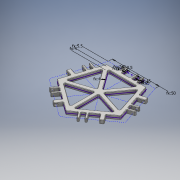
# Autodesk Inventor part: pentagon
Saved by Autodesk Inventor 2016 (Build 200138000, 138)
## iProperties
Created: 2016-11-12
Part Number: pentagon
Material: Generic
Document SubType Name: Modeling
Designer: Chris
Density: 1 g/cm^3
Appearance: Default
Author: Chris
Autodesk Inventor part; units mm, degrees
ref_plane "YZ Plane" through (0, 0, 0) normal (1, 0, 0) x (0, 1, 0)
ref_plane "XZ Plane" through (0, 0, 0) normal (0, 1, 0) x (-1, 0, 0)
ref_plane "XY Plane" through (0, 0, 0) normal (0, 0, 1) x (1, 0, 0)
sketch "Sketch1" plane through (0, 0, 0) normal (0, 0, 1) x (1, 0, 0)
  line L0 (25, 34.409548) -> (40.45085, -13.143278) construction
  line L1 (40.45085, -13.143278) -> (0, -42.53254) construction
  line L2 (0, -42.53254) -> (-40.45085, -13.143278) construction
  line L3 (-40.45085, -13.143278) -> (-25, 34.409548) construction
  line L4 (-25, 34.409548) -> (25, 34.409548) construction
  line L5 (21.004016, 28.909548) -> (33.985212, -11.042465)
  line L6 (33.985212, -11.042465) -> (0, -35.734167)
  line L7 (0, -35.734167) -> (-33.985212, -11.042465)
  line L8 (-33.985212, -11.042465) -> (-21.004016, 28.909548)
  line L9 (-21.004016, 28.909548) -> (21.004016, 28.909548)
  line L10 (0, -35.734167) -> (0, 0) construction
  line L11 (-18.097846, 24.909548) -> (-29.28293, -9.514601)
  line L12 (-29.28293, -9.514601) -> (0, -30.789895)
  line L13 (0, -30.789895) -> (29.28293, -9.514601)
  line L14 (29.28293, -9.514601) -> (18.097846, 24.909548)
  line L15 (18.097846, 24.909548) -> (-18.097846, 24.909548)
  line L16 (-7.5, 34.409548) -> (7.5, 34.409548) construction
  line L17 (3.475, 34.409548) -> (5.475, 34.409548) construction
  line L18 (5.475, 34.409548) -> (9.525, 34.409548) construction
  line L19 (11.525, 34.409548) -> (9.525, 34.409548) construction
  line L20 (-9.475, 34.409548) -> (-5.525, 34.409548) construction
  line L21 (-9.475, 28.909548) -> (-5.525, 28.909548)
  line L22 (-5.525, 28.909548) -> (-5.525, 36.409548)
  line L23 (-5.525, 36.409548) -> (-9.475, 36.409548)
  line L24 (-9.475, 36.409548) -> (-9.475, 28.909548)
  line L25 (3.475, 36.409548) -> (5.475, 36.409548)
  line L26 (5.475, 36.409548) -> (5.475, 28.909548)
  line L27 (5.475, 28.909548) -> (3.475, 28.909548)
  line L28 (3.475, 28.909548) -> (3.475, 36.409548)
  line L29 (9.525, 36.409548) -> (11.525, 36.409548)
  line L30 (11.525, 36.409548) -> (11.525, 28.909548)
  line L31 (11.525, 28.909548) -> (9.525, 28.909548)
  line L32 (9.525, 28.909548) -> (9.525, 36.409548)
  line L33 (-9.475, 34.409548) -> (-8.975, 34.409548)
  line L34 (-9.475, 34.409548) -> (-9.475, 35.909548)
  line L35 (-6.025, 34.409548) -> (-5.525, 34.409548)
  line L36 (-5.525, 34.409548) -> (-5.525, 35.909548)
  arc A0 (-8.975, 34.409548) -> (-9.475, 35.909548) centre (-11.475, 34.409548) ccw
  arc A1 (-5.525, 35.909548) -> (-6.025, 34.409548) centre (-3.525, 34.409548) ccw
  line L37 (5.475, 35.909548) -> (5.475, 34.409548)
  line L38 (5.475, 34.409548) -> (5.975, 34.409548)
  line L39 (9.525, 35.909548) -> (9.525, 34.409548)
  line L40 (9.525, 34.409548) -> (9.025, 34.409548)
  arc A2 (5.975, 34.409548) -> (5.475, 35.909548) centre (3.475, 34.409548) ccw
  arc A3 (9.525, 35.909548) -> (9.025, 34.409548) centre (11.525, 34.409548) ccw
  line L41 (-18.097846, 24.909548) -> (0, 0) construction
  line L42 (-29.28293, -9.514601) -> (0, 0) construction
  line L43 (18.097846, 24.909548) -> (0, 0) construction
  line L44 (29.28293, -9.514601) -> (0, 0) construction
  line L45 (0, 0) -> (-23.690388, 7.697474) construction
  line L46 (0, 24.909548) -> (0, 0) construction
  line L47 (0, 0) -> (23.690388, 7.697474) construction
  line L48 (0, 0) -> (14.641465, -20.152248) construction
  line L49 (-14.641465, -20.152248) -> (0, 0) construction
  line L50 (-18.861778, 22.558407) -> (-3.236068, 1.051462)
  line L51 (-3.236068, 1.051462) -> (-28.518998, -7.16346)
  line L52 (-15.62571, 24.909548) -> (0, 3.402603)
  line L53 (15.62571, 24.909548) -> (0, 3.402603)
  line L54 (18.861778, 22.558407) -> (3.236068, 1.051462)
  line L55 (28.518998, -7.16346) -> (3.236068, 1.051462)
  line L56 (27.28293, -10.967686) -> (2, -2.752764)
  line L57 (2, -2.752764) -> (2, -29.33681)
  line L58 (-2, -29.33681) -> (-2, -2.752764)
  line L59 (-2, -2.752764) -> (-27.28293, -10.967686)
  point P0 (0, 34.409548)
  dimension "d0" = 50
  dimension "d1" = 5.5
  dimension "d2" = 4
  dimension "d3" = 15
  dimension "d4" = 2
  dimension "d5" = 4.05
  dimension "d6" = 3.95
  dimension "d9" = 4
  dimension "d12" = 3
  dimension "d13" = 0.5
  dimension "d26" = 4
  constraints: 120 end point, 33 point on line, 16 parallel, 10 equal length, 9 midpoint, 8 horizontal, 8 point on circle, 7 coincident, 6 perpendicular, 5 vertical, 4 centre point, 2 collinear, 2 equal radius, 19 other
  measures "d0" distance of L3.end L0.start
  measures "d1" distance between parallel lines of L9 L4
  measures "d2" distance between parallel lines of L9 L15
  measures "d3" distance of L16.start L16.end
  measures "d4" distance of L19.start L18.end
  measures "d5" distance of L17.end L18.end
  measures "d6" distance of L20.start L20.end
  measures "d9" diameter of L23 L4
  measures "d12" diameter of L34.end L33
  measures "d13" distance of L20.start L33.end
  measures "d26" distance between parallel lines of L52 L50
extrude "Extrusion3" add sketch "Sketch1" along normal mid plane 4 contours L5 L6 L7 L8 L9 | L15 L52 L53 L14 L54 L55 L13 L56 L57 L12 L58 L59 L11 L51 L50
extrude "Extrusion2" add sketch "Sketch1" along normal mid plane 4 contours L9 L32 L29 L30 | L9 L28 L25 L26 | L24 L33 A0 L23 L22 A1 L35 L9 | L24 A0 L33 | L35 A1 L22
revolve "Revolution1" add sketch "Sketch1" angle 360 about axis through (-25, 34.409548, 0) along (1, 0, 0) contours L40 A3 L32 | L26 A2 L38
revolve "Revolution3" cut sketch "Sketch1" angle 360 about axis through (-9.475, 34.409548, 0) along (1, 0, 0) contours L24 A0 L33 | L35 A1 L22
fillet "Fillet5" radius 1 20 edges at (-21.004, 28.9095, 0) (21.004, 28.9095, 0) (33.9852, -11.0425, 0) (0, -35.7342, 0) (-33.9852, -11.0425, 0) (-18.8618, 22.5584, 0) (-15.6257, 24.9095, 0) (15.6257, 24.9095, 0) (0, 3.4026, 0) (-3.2361, 1.0515, 0) (-2, -2.7528, 0) (2, -2.7528, 0) (3.2361, 1.0515, 0) (-28.519, -7.1635, 0) (-27.2829, -10.9677, 0) (-2, -29.3368, 0) (2, -29.3368, 0) (27.2829, -10.9677, 0) (28.519, -7.1635, 0) (18.8618, 22.5584, 0)
pattern_circular "Circular Pattern1" count 5 over 360 about axis through (0, 0, -10) along (0, 0, 1) of "Extrusion2", "Revolution1", "Revolution3"
fillet "Fillet4" radius 0.75 60 edges at (-30.7249, -22.6817, 0) (-29.1069, -23.8573, 0) (-25.8304, -26.2378, 0) (-24.2123, -27.4134, 0) (-16.9312, -32.7035, 0) (-13.7356, -35.0252, 0) (29.0664, -23.8867, 0) (25.8708, -26.2084, 0) (18.5897, -31.4985, 0) (16.9716, -32.6741, 0) (13.6951, -35.0546, 0) (12.0771, -36.2302, 0) (38.189, 0.2902, 0) (37.5709, 2.1924, 0) (36.3194, 6.0441, 0) (35.7014, 7.9462, 0) (32.9202, 16.5058, 0) (31.6996, 20.2624, 0) (-9.475, 36.4095, 0) (-5.525, 36.4095, 0) (3.475, 36.4095, 0) (5.475, 36.4095, 0) (9.525, 36.4095, 0) (11.525, 36.4095, 0) (-31.6842, 20.31, 0) (-31.0661, 22.2121, 0) (-32.9357, 16.4582, 0) (-33.5537, 14.5561, 0) (-36.3349, 5.9966, 0) (-37.5555, 2.2399, 0) (-9.475, 28.9095, 0) (-5.525, 28.9095, 0) (3.475, 28.9095, 0) (5.475, 28.9095, 0) (9.525, 28.9095, 0) (11.525, 28.9095, 0) (24.5667, 17.9448, 0) (25.7873, 14.1881, 0) (28.5684, 5.6286, 0) (29.1865, 3.7265, 0) (30.438, -0.1253, 0) (31.056, -2.0274, 0) (24.658, -17.8191, 0) (21.4624, -20.1408, 0) (14.1813, -25.4309, 0) (12.5632, -26.6064, 0) (9.2867, -28.987, 0) (7.6687, -30.1625, 0) (-9.3272, -28.9576, 0) (-12.5228, -26.6358, 0) (-21.422, -20.1702, 0) (-19.8039, -21.3458, 0) (-26.3165, -16.6141, 0) (-24.6985, -17.7897, 0) (-30.4226, -0.0777, 0) (-29.2019, 3.679, 0) (-26.4208, 12.2385, 0) (-25.8027, 14.1406, 0) (-24.5512, 17.9924, 0) (-23.9332, 19.8945, 0)
chamfer "Chamfer2" distance 0.4 angle 45 260 edges at (-15.2512, 28.9095, 2) (-20.8653, 28.7186, 2) (-22.465, 24.4132, 2) (-24.0742, 20.1713, 2) (-27.4997, 21.0533, 2) (-30.9251, 21.9353, 2) (-31.3751, 21.261, 2) (-31.4074, 20.451, 2) (-28.1177, 19.1512, 2) (-24.828, 17.8513, 2) (-25.177, 16.0665, 2) (-25.9438, 14.4174, 2) (-29.3692, 15.2994, 2) (-32.7946, 16.1814, 2) (-33.2447, 15.5071, 2) (-33.2769, 14.6971, 2) (-29.9872, 13.3973, 2) (-26.6976, 12.0974, 2) (-27.8114, 7.9587, 2) (-29.343, 3.9558, 2) (-32.7684, 4.8378, 2) (-36.1938, 5.7198, 2) (-36.9452, 4.1182, 2) (-37.2787, 2.3809, 2) (-33.989, 1.0811, 2) (-30.6994, -0.2188, 2) (-32.2075, -5.5712, 2) (-33.7607, -10.9695, 2) (-30.1604, -13.8214, 2) (-26.6234, -16.6627, 2) (-28.5207, -19.6479, 2) (-30.4181, -22.6331, 2) (-29.9159, -23.2695, 2) (-29.1555, -23.5505, 2) (-26.9027, -20.8235, 2) (-24.6499, -18.0965, 2) (-23.0602, -18.9799, 2) (-21.7288, -20.2188, 2) (-23.6262, -23.204, 2) (-25.5235, -26.1892, 2) (-25.0213, -26.8256, 2) (-24.2609, -27.1066, 2) (-22.0081, -24.3796, 2) (-19.7553, -21.6526, 2) (-16.1634, -23.9908, 2) (-12.8296, -26.6844, 2) (-14.727, -29.6696, 2) (-16.6243, -32.6549, 2) (-15.3334, -33.8643, 2) (-13.7842, -34.7184, 2) (-11.5314, -31.9914, 2) (-9.2786, -29.2644, 2) (-4.6541, -32.3528, 2) (0, -35.4981, 2) (3.8249, -32.9552, 2) (7.6201, -30.4694, 2) (9.8729, -33.1964, 2) (12.1257, -35.9233, 2) (12.8861, -35.6424, 2) (13.3883, -35.006, 2) (11.4909, -32.0208, 2) (9.5936, -29.0356, 2) (10.925, -27.7967, 2) (12.5146, -26.9133, 2) (14.7674, -29.6403, 2) (17.0202, -32.3672, 2) (17.7806, -32.0863, 2) (18.2828, -31.4499, 2) (16.3855, -28.4647, 2) (14.4881, -25.4795, 2) (17.8218, -22.7858, 2) (21.4138, -20.4476, 2) (23.6666, -23.1746, 2) (25.9194, -25.9016, 2) (27.4686, -25.0476, 2) (28.7596, -23.8381, 2) (26.8622, -20.8529, 2) (24.9649, -17.8676, 2) (29.3311, -14.4239, 2) (33.7607, -10.9695, 2) (32.5242, -6.5461, 2) (31.3328, -2.1684, 2) (34.6225, -0.8686, 2) (37.9122, 0.4313, 2) (37.8799, 1.2413, 2) (37.4299, 1.9156, 2) (34.0045, 1.0335, 2) (30.579, 0.1515, 2) (29.8122, 1.8006, 2) (29.4633, 3.5855, 2) (32.7529, 4.8853, 2) (36.0426, 6.1852, 2) (36.0104, 6.9952, 2) (35.5603, 7.6694, 2) (32.1349, 6.7874, 2) (28.7095, 5.9054, 2) (27.1779, 9.9084, 2) (26.0641, 14.0471, 2) (29.3538, 15.3469, 2) (32.6434, 16.6468, 2) (-15.2512, 28.9095, -2) (-9.6947, 29.1292, -2) (-9.475, 32.6595, -2) (-9.2553, 36.1899, -2) (-7.5, 36.4095, -2) (-5.7447, 36.1899, -2) (-5.525, 32.6595, -2) (-5.3053, 29.1292, -2) (-1.025, 28.9095, -2) (3.2553, 29.1292, -2) (3.475, 32.6595, -2) (3.6947, 36.1899, -2) (4.475, 36.4095, -2) (5.2553, 36.1899, -2) (5.475, 32.6595, -2) (5.6947, 29.1292, -2) (7.5, 28.9095, -2) (9.3053, 29.1292, -2) (9.525, 32.6595, -2) (9.7447, 36.1899, -2) (10.525, 36.4095, -2) (11.3053, 36.1899, -2) (11.525, 32.6595, -2) (11.7447, 29.1292, -2) (16.2762, 28.9095, -2) (20.8653, 28.7186, -2) (22.7817, 23.4383, -2) (24.7077, 18.2216, -2) (28.1331, 19.1036, -2) (31.5586, 19.9856, -2) (32.3099, 18.3841, -2) (32.6434, 16.6468, -2) (29.3538, 15.3469, -2) (26.0641, 14.0471, -2) (27.1779, 9.9084, -2) (28.7095, 5.9054, -2) (32.1349, 6.7874, -2) (35.5603, 7.6694, -2) (36.0104, 6.9952, -2) (36.0426, 6.1852, -2) (32.7529, 4.8853, -2) (29.4633, 3.5855, -2) (29.8122, 1.8006, -2) (30.579, 0.1515, -2) (34.0045, 1.0335, -2) (37.4299, 1.9156, -2) (37.8799, 1.2413, -2) (37.9122, 0.4313, -2) (34.6225, -0.8686, -2) (31.3328, -2.1684, -2) (32.5242, -6.5461, -2) (33.7607, -10.9695, -2) (29.3311, -14.4239, -2) (24.9649, -17.8676, -2) (26.8622, -20.8529, -2) (28.7596, -23.8381, -2) (27.4686, -25.0476, -2) (25.9194, -25.9016, -2) (23.6666, -23.1746, -2) (21.4138, -20.4476, -2) (17.8218, -22.7858, -2) (14.4881, -25.4795, -2) (16.3855, -28.4647, -2) (18.2828, -31.4499, -2) (17.7806, -32.0863, -2) (17.0202, -32.3672, -2) (14.7674, -29.6403, -2) (12.5146, -26.9133, -2) (10.925, -27.7967, -2) (9.5936, -29.0356, -2) (11.4909, -32.0208, -2) (13.3883, -35.006, -2) (12.8861, -35.6424, -2) (12.1257, -35.9233, -2) (9.8729, -33.1964, -2) (7.6201, -30.4694, -2) (3.8249, -32.9552, -2) (0, -35.4981, -2) (-4.6541, -32.3528, -2) (-9.2786, -29.2644, -2) (-11.5314, -31.9914, -2) (-13.7842, -34.7184, -2) (-15.3334, -33.8643, -2) (-16.6243, -32.6549, -2) (-14.727, -29.6696, -2) (-12.8296, -26.6844, -2) (-16.1634, -23.9908, -2) (-19.7553, -21.6526, -2) (-22.0081, -24.3796, -2) (-24.2609, -27.1066, -2) (-25.0213, -26.8256, -2) (-25.5235, -26.1892, -2) (-23.6262, -23.204, -2) (-21.7288, -20.2188, -2) (-23.0602, -18.9799, -2) (-24.6499, -18.0965, -2) (-26.9027, -20.8235, -2) (-29.1555, -23.5505, -2) (-29.9159, -23.2695, -2) (-30.4181, -22.6331, -2) (7.6406, 13.9189, -2) (14.5541, 24.3635, -2) (0, 24.9095, -2) (-14.5541, 24.3635, -2) (-7.6406, 13.9189, -2) (0, 4.1039, -2) (7.6406, 13.9189, 2) (0, 4.1039, 2) (-7.6406, 13.9189, 2) (-14.5541, 24.3635, 2) (0, 24.9095, 2) (14.5541, 24.3635, 2) (-3.903, 1.2682, -2) (-15.5988, -2.9654, -2) (-27.6686, -6.313, -2) (-23.6904, 7.6975, -2) (-18.6736, 21.3705, -2) (-10.8766, 11.5678, -2) (-3.903, 1.2682, 2) (-10.8766, 11.5678, 2) (-18.6736, 21.3705, 2) (-23.6904, 7.6975, 2) (-27.6686, -6.313, 2) (-15.5988, -2.9654, 2) (-2.4122, -3.3201, -2) (-2, -15.7517, -2) (-2.546, -28.2652, -2) (-14.6415, -20.1522, -2) (-26.095, -11.1558, -2) (-14.3627, -6.7696, -2) (-2.4122, -3.3201, 2) (-14.3627, -6.7696, 2) (-26.095, -11.1558, 2) (-14.6415, -20.1522, 2) (-2.546, -28.2652, 2) (-2, -15.7517, 2) (2.4122, -3.3201, -2) (14.3627, -6.7696, -2) (26.095, -11.1558, -2) (14.6415, -20.1522, -2) (2.546, -28.2652, -2) (2, -15.7517, -2) (2.4122, -3.3201, 2) (2, -15.7517, 2) (2.546, -28.2652, 2) (14.6415, -20.1522, 2) (26.095, -11.1558, 2) (14.3627, -6.7696, 2) (3.903, 1.2682, -2) (10.8766, 11.5678, -2) (18.6736, 21.3705, -2) (23.6904, 7.6975, -2) (27.6686, -6.313, -2) (15.5988, -2.9654, -2) (3.903, 1.2682, 2) (15.5988, -2.9654, 2) (27.6686, -6.313, 2) (23.6904, 7.6975, 2) (18.6736, 21.3705, 2) (10.8766, 11.5678, 2)
equation "\"d0\" = sidelength"
equation "\"d1\" = springlength"
equation "\"d2\" = diam"
equation "\"d3\" = matespace"
equation "\"d4\" = springwidth"
equation "\"d5\" = fingerwidth + 0.5 * tolerance"
equation "\"d6\" = fingerwidth - 0.5 * tolerance"
equation "\"d9\" = diam"
equation "\"d12\" = dentdiam"
equation "\"d13\" = dent"
equation "\"d10\" = diam"
equation "\"sidelength\" = 50"
equation "\"diam\" = 4"
equation "\"dent\" = 0.5"
equation "\"dentdiam\" = 3"
equation "\"tolerance\" = 0.1"
equation "\"fingerwidth\" = 4"
equation "\"springwidth\" = 2"
equation "\"matespace\" = 15"
equation "\"springlength\" = 5.5"
body "Solid1"
body "Solid2"
